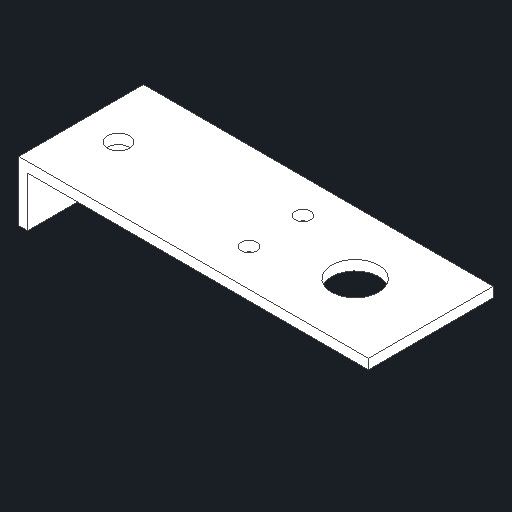
# Autodesk Inventor part: Top Connecter 1
Saved by Autodesk Inventor 2026.1 (Build 301233020, 233B)
## iProperties
Created: 2025-11-25
Part Number: Top Connecter 1
Material: Generic
Document SubType Name: Modeling
Designer: sarab
Density: 1 g/cm^3
Appearance: Default
Author: sarab
Autodesk Inventor part; units mm, degrees
ref_plane "YZ Plane" through (0, 0, 0) normal (1, 0, 0) x (0, 1, 0)
ref_plane "XZ Plane" through (0, 0, 0) normal (0, 1, 0) x (-1, 0, 0)
ref_plane "XY Plane" through (0, 0, 0) normal (0, 0, 1) x (1, 0, 0)
sketch "Sketch1" plane through (0, 0, 0) normal (0, 0, 1) x (1, 0, 0)
  line L0 (0, 0) -> (0, 15.6)
  line L1 (0, 15.6) -> (91, 15.6)
  line L2 (91, 15.6) -> (91, 13)
  line L3 (0, 0) -> (2.305, 0)
  line L4 (2.305, 0) -> (2.305, 13)
  line L5 (2.305, 13) -> (91, 13)
  constraints: 12 end point, 3 perpendicular, 2 vertical, 1 horizontal
extrude "Extrusion1" add sketch "Sketch1" along normal blind 32.462
sketch "Sketch2" plane through (0, 15.6, 0) normal (0, 1, 0) x (1, 0, 0)
  line L0 (0, 0) -> (0, -32.462) projected
  line L1 (2.305, -32.462) -> (91, -32.462) projected
  circle A0 centre (9.701, -16.231) radius 2.861
  circle A1 centre (71.299, -16.231) radius 6.1315
  circle A2 centre (50.2582, -22.803) radius 2
  circle A3 centre (50.2582, -8.803) radius 2
  constraints: 4 centre point
extrude "Extrusion2" cut sketch "Sketch2" against normal blind 32.462
body "Solid1"
